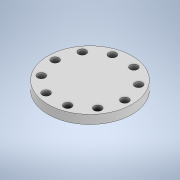
# Autodesk Inventor part: Крышка стакана
Saved by Autodesk Inventor 2021 (Build 250183000, 183)
## iProperties
Created: 2020-11-15
Part Number: Крышка стакана
Material: Типовые
Document SubType Name: Modeling
Designer: Тимоха
Density: 1 g/cm^3
Appearance: По умолчанию
Author: Тимоха
Autodesk Inventor part; units mm, degrees
ref_plane "YZ Plane" through (0, 0, 0) normal (1, 0, 0) x (0, 1, 0)
ref_plane "XZ Plane" through (0, 0, 0) normal (0, 1, 0) x (-1, 0, 0)
ref_plane "XY Plane" through (0, 0, 0) normal (0, 0, 1) x (1, 0, 0)
sketch "Эскиз1" plane through (0, 0, 0) normal (0, 0, 1) x (1, 0, 0)
  line L0 (0, 0) -> (78, 0)
  line L1 (78, 0) -> (78, 24)
  line L2 (78, 24) -> (120, 24)
  line L3 (120, 24) -> (120, 49)
  line L4 (120, 49) -> (0, 49)
  line L5 (78, 0) -> (71, 0)
  line L6 (71, 0) -> (68.195, 11.1488)
  line L7 (68.195, 11.1488) -> (68.195, 20.9431)
  line L8 (68.195, 20.9431) -> (0, 20.9431)
  line L9 (0, 49) -> (0, 20.9431)
  dimension "d0" = 78
  dimension "d1" = 24
  dimension "d2" = 42
  dimension "d3" = 25
  dimension "d4" = 7
  constraints: 20 end point, 3 perpendicular, 3 vertical, 2 horizontal, 1 point on line
  measures "d0" distance of L0.start L0.end
  measures "d1" distance of L0.end L1.end
  measures "d2" distance of L1.end L2.end
  measures "d3" distance of L2.end L3.end
  measures "d4" distance of L0.end L5.end
revolve "Вращение1" add sketch "Эскиз1" angle 360 about axis through (0, 49, 0) along (0, -1, 0)
sketch "Эскиз2" plane through (0, 49, 0) normal (0, 1, 0) x (1, 0, 0)
  circle A0 centre (0, 0) radius 120 projected
  line L0 (120, 0) -> (99.5, 0)
  point P0 (0, 0)
  dimension "d7" = 20.5
  constraints: 2 end point, 1 horizontal, 1 horizontal alignment, 1 other
  measures "d7" distance of L0.start L0.end
hole "Отверстие1" at (99.5, 49, 0) direction (0, -1, 0) diameter 22 end through all
pattern_circular "Круговой массив1" count 10 over 360 about axis through (0, 16.0459, 0) along (0, -1, 0) of "Отверстие1"
